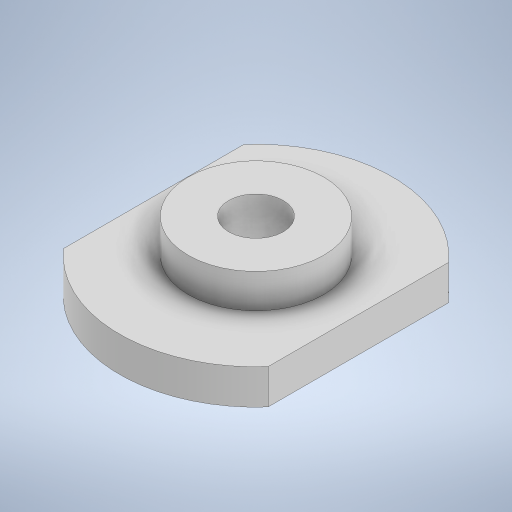
# Autodesk Inventor part: C-Channel Spacer M3
Saved by Autodesk Inventor 2024 (Build 280153020, 153B)
## iProperties
Created: 2023-12-18
Part Number: C-Channel Spacer M3
Material: Generic
Document SubType Name: Modeling
Designer: scottst
Density: 1 g/cm^3
Appearance: Default
Author: scottst
Autodesk Inventor part; units mm, degrees
ref_plane "YZ Plane" through (0, 0, 0) normal (1, 0, 0) x (0, 1, 0)
ref_plane "XZ Plane" through (0, 0, 0) normal (0, 1, 0) x (-1, 0, 0)
ref_plane "XY Plane" through (0, 0, 0) normal (0, 0, 1) x (1, 0, 0)
sketch "Sketch1" plane through (0, 0, 0) normal (0, 1, 0) x (-1, 0, 0)
  circle A0 centre (0, 0) radius 3.975
  circle A1 centre (0, 0) radius 1.6
  circle A2 centre (0, 0) radius 8
  dimension "d0" = 7.95
  dimension "d1" = 3.2
  dimension "d2" = 16
  constraints: 3 centre point, 3 coincident
  measures "d0" diameter of A0
  measures "d1" diameter of A1
  measures "d2" diameter of A2
extrude "Extrusion1" add sketch "Sketch1" along normal blind 2 contours A0
extrude "Extrusion2" add sketch "Sketch1" against normal blind 3.8 contours A0 | A2
sketch "Sketch3" plane through (0, -3.8, 0) normal (0, -1, 0) x (1, 0, 0)
  line L0 (8, 0) -> (6, 0) construction
  line L1 (6, 0) -> (6, -6.7165)
  line L2 (6, 0) -> (6, 8)
  line L3 (6, 8) -> (11.3207, 8)
  line L4 (11.3207, 8) -> (13.7407, -4.0569)
  line L5 (13.7407, -4.0569) -> (10.7642, -6.413)
  line L6 (10.7642, -6.413) -> (6, -6.7165)
  dimension "d11" = 2
  constraints: 14 end point, 2 perpendicular, 1 horizontal, 1 vertical
  measures "d11" distance of L0.start L0.end
extrude "Extrusion4" cut sketch "Sketch3" against normal blind 6.75
mirror "Mirror1" about plane through (0, 0, 0) normal (1, 0, 0) of "Extrusion4"
sketch "Sketch4" plane through (0, -3.8, 0) normal (0, -1, 0) x (1, 0, 0)
  line L0 (-6, 5.2915) -> (-6, -5.2915) projected
  arc A0 (-6, -5.2915) -> (6, -5.2915) centre (0, 0) ccw projected
  line L1 (6, -5.2915) -> (6, 5.2915) projected
  arc A1 (6, 5.2915) -> (-6, 5.2915) centre (0, 0) ccw projected
  circle A2 centre (0, 0) radius 1.6 projected
extrude "Extrusion5" cut sketch "Sketch4" against normal blind 1.75
body "Solid1"
